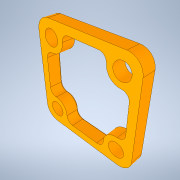
# Autodesk Inventor part: Проставка датчика
Saved by Autodesk Inventor 2021.1 (Build 251245010, 245A)
## iProperties
Created: 2026-05-20
Part Number: Проставка датчика
Material: Типовые
Document SubType Name: Modeling
Designer: Андрей Тарасов
Density: 1 g/cm^3
Appearance: По умолчанию
Author: Андрей Тарасов
Autodesk Inventor part; units mm, degrees
ref_plane "YZ Plane" through (0, 0, 0) normal (1, 0, 0) x (0, 1, 0)
ref_plane "XZ Plane" through (0, 0, 0) normal (0, 1, 0) x (-1, 0, 0)
ref_plane "XY Plane" through (0, 0, 0) normal (0, 0, 1) x (1, 0, 0)
sketch "Эскиз1" plane through (0, 0, 0) normal (0, 0, 1) x (1, 0, 0)
  line L0 (8.5, -11.5) -> (-8.5, -11.5)
  line L1 (-11.5, -8.5) -> (-11.5, 8.5)
  line L2 (-8.5, 11.5) -> (8.5, 11.5)
  line L3 (11.5, 8.5) -> (11.5, -8.5)
  line L4 (11.5, -11.5) -> (-11.5, 11.5) construction
  line L5 (-11.5, -11.5) -> (11.5, 11.5) construction
  line L6 (8, -8) -> (-8, -8) construction
  line L7 (-8, -8) -> (-8, 8) construction
  line L8 (-8, 8) -> (8, 8) construction
  line L9 (8, 8) -> (8, -8) construction
  line L10 (8, -8) -> (-8, 8) construction
  line L11 (-8, -8) -> (8, 8) construction
  circle A0 centre (-8, 8) radius 1.75
  circle A1 centre (8, 8) radius 1.75
  circle A2 centre (-8, -8) radius 1.75
  circle A3 centre (8, -8) radius 1.75
  arc A4 (-8.5, 11.5) -> (-11.5, 8.5) centre (-8.5, 8.5) ccw
  arc A5 (11.5, 8.5) -> (8.5, 11.5) centre (8.5, 8.5) ccw
  arc A6 (-11.5, -8.5) -> (-8.5, -11.5) centre (-8.5, -8.5) ccw
  arc A7 (8.5, -11.5) -> (11.5, -8.5) centre (8.5, -8.5) ccw
  line L12 (-9.75, 9.75) -> (9.75, 9.75)
  line L13 (9.75, 9.75) -> (9.75, -9.75)
  line L14 (9.75, -9.75) -> (-9.75, -9.75)
  line L15 (-9.75, -9.75) -> (-9.75, 9.75)
  circle A8 centre (-8, 8) radius 3
  circle A9 centre (8, 8) radius 3
  circle A10 centre (8, -8) radius 3
  circle A11 centre (-8, -8) radius 3
  point P0 (0, 0)
  point P1 (0, 0)
  point P2 (-5.5633, 9.75)
  point P3 (5.5633, 9.75)
  point P4 (9.75, 5.5633)
  point P5 (9.75, -5.5633)
  point P6 (5.5633, -9.75)
  point P7 (-5.5633, -9.75)
  point P8 (-9.75, -5.5633)
  point P9 (-9.75, 5.5633)
  dimension "d0" = 23
  dimension "d2" = 16
  dimension "d4" = 3.5
  dimension "d5" = 3
  dimension "d8" = 6
  constraints: 32 end point, 12 centre point, 10 point on line, 10 tangent, 9 coincident, 9 equal radius, 8 point on circle, 6 parallel, 5 perpendicular, 4 midpoint, 3 horizontal
  measures "d0" distance of L4.end L5.end
  measures "d2" distance of L7.end L8.end
  measures "d4" diameter of A0
  measures "d5" radius of A4
  measures "d8" diameter of A8
extrude "Выдавливание1" add sketch "Эскиз1" along normal blind 3.2 contours L0 A6 L1 A4 L2 A5 L3 A7 | A0 L12 A8 L15 | A0 L15 L12 | L12 L15 A8 | A9 L13 L12 | L12 A1 L13 A9 | A11 L14 A2 L15 | L15 L14 A11 | L12 L13 A1 | A2 L14 L15 | A10 L14 L13 | L13 A3 L14 A10 | L13 L14 A3
fillet "Сопряжение1" radius 1.6 8 edges at (5.5633, 9.75, 1.6) (-5.5633, 9.75, 1.6) (-9.75, 5.5633, 1.6) (-9.75, -5.5633, 1.6) (-5.5633, -9.75, 1.6) (5.5633, -9.75, 1.6) (9.75, -5.5633, 1.6) (9.75, 5.5633, 1.6)
chamfer "Фаска1" distance 0.4 angle 45 20 edges at (-9.75, -8, 0) (6.25, -8, 0) (6.25, 8, 0) (-9.75, 8, 0) (0, 9.75, 0) (5.8787, 5.8787, 0) (9.75, 0, 0) (5.8787, -5.8787, 0) (0, -9.75, 0) (-5.8787, -5.8787, 0) (-9.75, 0, 0) (-5.8787, 5.8787, 0) (0, 11.5, 0) (-10.6213, 10.6213, 0) (-11.5, 0, 0) (-10.6213, -10.6213, 0) (0, -11.5, 0) (10.6213, -10.6213, 0) (11.5, 0, 0) (10.6213, 10.6213, 0)
